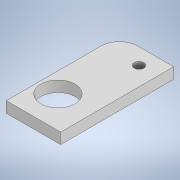
# Autodesk Inventor part: corner spacers
Saved by Autodesk Inventor 2021 (Build 250183000, 183)
## iProperties
Created: 2020-08-18
Part Number: corner spacers
Material: Generic
Document SubType Name: Modeling
Designer: jgray
Density: 1 g/cm^3
Appearance: Default
Author: jgray
Autodesk Inventor part; units mm, degrees
ref_plane "YZ Plane" through (0, 0, 0) normal (1, 0, 0) x (0, 1, 0)
ref_plane "XZ Plane" through (0, 0, 0) normal (0, 1, 0) x (-1, 0, 0)
ref_plane "XY Plane" through (0, 0, 0) normal (0, 0, 1) x (1, 0, 0)
sketch "Sketch1" plane through (0, 0, 0) normal (0, 1, 0) x (-1, 0, 0)
  line L0 (0, 0) -> (25, 0)
  line L1 (25, 0) -> (25, -43.5)
  line L2 (16.5, -52) -> (0, -52)
  line L3 (0, -52) -> (0, 0)
  arc A0 (16.5, -52) -> (25, -43.5) centre (16.5, -43.5) ccw
  circle A1 centre (15.8, -14.55) radius 7.875
  circle A2 centre (8.5, -44.55) radius 2.2
  line L4 (5, 10.2052) -> (5, -72.053) construction
  point P0 (25, -52)
  dimension "d0" = 25
  dimension "d1" = 52
  dimension "d2" = 8.5
  dimension "d3" = 15.75
  dimension "d4" = 4.4
  dimension "d5" = 16.5
  dimension "d6" = 7.45
  dimension "d7" = 20
  dimension "d8" = 9.2
  dimension "d9" = 30
  constraints: 10 end point, 3 centre point, 2 parallel, 2 point on circle, 2 point on line, 2 tangent, 1 horizontal, 1 perpendicular, 1 vertical
  measures "d0" distance of point (25, -52) L2.end
  measures "d1" distance of L0.end point (25, -52)
  measures "d2" radius of A0
  measures "d3" diameter of A1
  measures "d4" diameter of A2
  measures "d5" distance from line of L1 A2.centre
  measures "d6" distance from line of L2 A2.centre
  measures "d7" distance between parallel lines of L1 L4
  measures "d8" distance from line of A1.centre L1
  measures "d9" vertical distance of A2.centre A1.centre
extrude "Extrusion1" add sketch "Sketch1" along normal blind 5
body "Solid1"
